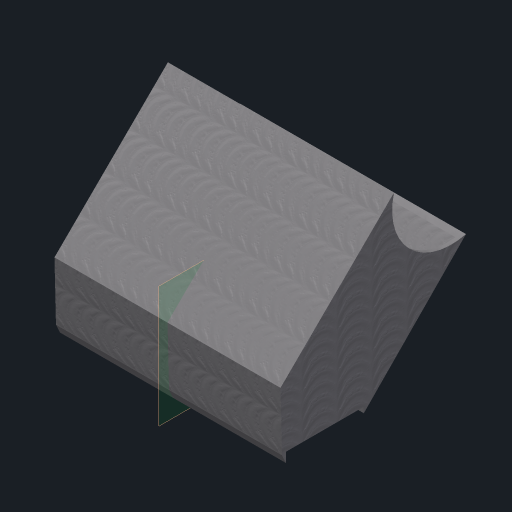
# Autodesk Inventor part: CANALETA_GUIA
Saved by Autodesk Inventor 2024.3 (Build 283343000, 343)
## iProperties
Created: 2024-07-12
Part Number: CANALETA_GUIA
Material: Steel, Mild, Welded
Document SubType Name: Modeling
Designer: Niler
Density: 7.85 g/cm^3
Appearance: Weld - Steel Mild
Author: Niler
Autodesk Inventor part; units mm, degrees
ref_plane "YZ Plane" through (0, 0, 0) normal (1, 0, 0) x (0, 1, 0)
ref_plane "XZ Plane" through (0, 0, 0) normal (0, 1, 0) x (-1, 0, 0)
ref_plane "XY Plane" through (0, 0, 0) normal (0, 0, 1) x (1, 0, 0)
sketch "Sketch1" plane through (0, 0, 0) normal (1, 0, 0) x (0, 1, 0)
  line L0 (42.8643, -50) -> (204.4541, -208.7035)
  line L1 (0, 0) -> (0, -50)
  line L2 (124.4924, 56.8774) -> (295.5459, -115.955)
  line L3 (122.4584, 51.8246) -> (292.042, -119.5226)
  line L4 (50, -50) -> (207.9576, -205.1362)
  line L5 (295.5459, -115.955) -> (204.4541, -208.7035)
  circle A0 centre (250, -162.3292) radius 10
  circle A1 centre (250, -162.3292) radius 76
  line L6 (124.4924, 56.8774) -> (-148.62, 50)
  line L7 (50, 50) -> (122.4584, 51.8246)
  line L8 (0, 0) -> (0, -77.5)
  line L9 (-50, 50) -> (50, 50)
  line L10 (50, 50) -> (50, -50)
  line L11 (50, -50) -> (-50, -50)
  line L12 (-50, -50) -> (-50, 50)
  line L13 (-50, 50) -> (50, -50) construction
  line L14 (50, 50) -> (-50, -50) construction
  line L15 (37.5556, 50) -> (48.6277, 54.967)
  point P0 (22.0043, 0)
  point P1 (259.821, -86.9665)
  point P2 (268.4835, -88.6111)
  point P3 (176.3565, -181.1077)
  point P4 (174.6769, -172.4499)
  point P5 (242.9929, -169.4637)
  point P6 (257.0071, -155.1947)
  dimension "d6" = 5
  dimension "d7" = 5
  dimension "d8" = 90
  dimension "d9" = 130
  dimension "d11" = 50
  dimension "d14" = 20
  dimension "d16" = 152
  dimension "d17" = 250
  dimension "d18" = 5
  dimension "d24" = 77.5
  dimension "d26" = 264
  dimension "d29" = 100
  dimension "d30" = 100
  constraints: 32 end point, 6 point on line, 5 parallel, 3 coincident, 3 midpoint, 2 centre point, 2 vertical, 1 horizontal, 1 horizontal alignment, 1 perpendicular
  measures "d6" distance between parallel lines of L3 L2
  measures "d7" distance between parallel lines of L0 L4
  measures "d8" angle of L5 L0
  measures "d9" distance of L2.end L0.end
  measures "d11" distance of L1.start L1.end
  measures "d14" diameter of A0
  measures "d16" diameter of A1
  measures "d17" distance from line of A0.centre L1
  measures "d18" distance between parallel lines of L6 L7
  measures "d24" distance of L1.start L8.end
  measures "d26" distance of A0.centre L8.end
  measures "d29" distance of L4.start L11.end
  measures "d30" distance of L7.start L4.start
extrude "Extrusion1" add sketch "Sketch1" against normal blind 280 contours L11 L4 A1 L0 | L9 L15 L6 L2 A1 L3 L7
extrude "Extrusion2" add sketch "Sketch1" along normal blind 5 contours L11 L4 A1 L0 | L10 L7 L3 A1 L4 | L9 L15 L6 L2 A1 L3 L7
ref_plane "Work Plane1" through (-140, 0, 0) normal (-1, 0, 0) x (0, 0, 1)
mirror "Mirror1" about plane through (-140, 0, 0) normal (-1, 0, 0) of "Extrusion2"
body "Solid1"
